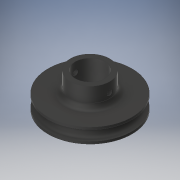
# Autodesk Inventor part: 0.5OD_Pulley
Saved by Autodesk Inventor 2019 (Build 230136000, 136)
## iProperties
Created: 2021-02-23
Part Number: 0.5OD_Pulley
Material: ABS Plastic
Document SubType Name: Modeling
Designer: zhanb
Density: 1.06 g/cm^3
Appearance: Smooth - Black
Author: zhanb
Autodesk Inventor part; units mm, degrees
ref_plane "YZ Plane" through (0, 0, 0) normal (1, 0, 0) x (0, 1, 0)
ref_plane "XZ Plane" through (0, 0, 0) normal (0, 1, 0) x (-1, 0, 0)
ref_plane "XY Plane" through (0, 0, 0) normal (0, 0, 1) x (1, 0, 0)
sketch "Sketch1" plane through (0, 0, 0) normal (1, 0, 0) x (0, 1, 0)
  line L0 (-2.3813, 13.5064) -> (-2.3813, 0) construction
  line L1 (-2.3813, 0) -> (0, 0) construction
  line L2 (2.3813, 0) -> (2.3813, 13.5064)
  line L3 (2.3813, 13.5064) -> (0, 13.5064)
  line L4 (-2.3813, 13.5064) -> (2.3813, 0) construction
  line L5 (-2.3813, 0) -> (2.3813, 13.5064) construction
  line L6 (0, 12.7) -> (0, 11.0871)
  line L7 (0, 11.0871) -> (0, 13.5064)
  line L8 (0, 13.5064) -> (-2.3813, 13.5064) construction
  line L9 (0, 0) -> (2.3813, 0)
  line L10 (0, 11.0871) -> (0, 0)
  arc A0 (0, 11.0871) -> (1.6129, 12.7) centre (0, 12.7) ccw
  line L11 (1.6129, 12.7) -> (1.6129, 13.5064)
  point P0 (0, 6.7532)
  point P1 (0, 6.7532)
  dimension "d2" = 1.6129
  dimension "d4" = 2.3813
  dimension "d5" = 0.8065
  dimension "d16" = 12.7
  constraints: 24 end point, 5 parallel, 4 vertical, 3 midpoint, 3 point on line, 2 perpendicular, 2 point on circle, 1 centre point, 1 tangent
  measures "d2" radius of A0
  measures "d4" distance of L2.end L3.end
  measures "d5" distance of L3.end L6.start
  measures "d16" distance of L1.end L6.start
revolve "Revolution1" add sketch "Sketch1" angle 360 about axis through (0, 0, 0) along (0, 1, 0) contours L9 L10 A0 L11 L3 L2
mirror "Mirror1" about plane through (0, 0, 11.0871) normal (0, -1, 0) of "Revolution1"
sketch "Sketch2" plane through (0, -2.3813, 0) normal (0, -1, 0) x (1, 0, 0)
  circle A0 centre (0, 0) radius 4.7625
  point P0 (0, 0)
  dimension "d7" = 9.525
  constraints: 1 centre point, 1 coincident
  measures "d7" diameter of A0
extrude "Extrusion1" cut sketch "Sketch2" against normal through all
sketch "Sketch3" plane through (0, 2.3813, 0) normal (0, 1, 0) x (1, 0, 0)
  circle A0 centre (0, 0) radius 4.7625 projected
  circle A1 centre (0, 0) radius 6.35
  dimension "d10" = 1.5875
  constraints: 1 centre point, 1 coincident
  measures "d10" radial gap between concentric circles of A0 A1
extrude "Extrusion2" add sketch "Sketch3" along normal blind 6.35
sketch "Sketch4" plane through (0, 0, 0) normal (1, 0, 0) x (0, 1, 0)
  circle A0 centre (5.5563, 0) radius 0.7937
  line L0 (8.7312, -6.35) -> (8.7313, 6.35) construction
  line L1 (2.3813, 6.35) -> (2.3812, -6.35) construction
  line L2 (8.7312, -6.35) -> (8.7313, 6.35) projected
  line L3 (2.3813, 6.35) -> (8.7312, -6.35) construction
  point P0 (0, 0)
  dimension "d13" = 1.5875
  constraints: 2 end point, 1 centre point, 1 coincident, 1 midpoint
  measures "d13" diameter of A0
extrude "Extrusion3" cut sketch "Sketch4" along normal through all both and the other way through all
fillet "Fillet1" radius 1.5875 1 edges at (-6.35, 2.3813, 0)
equation "\"d5\" = 0.5 * d2"
body "Solid1"
